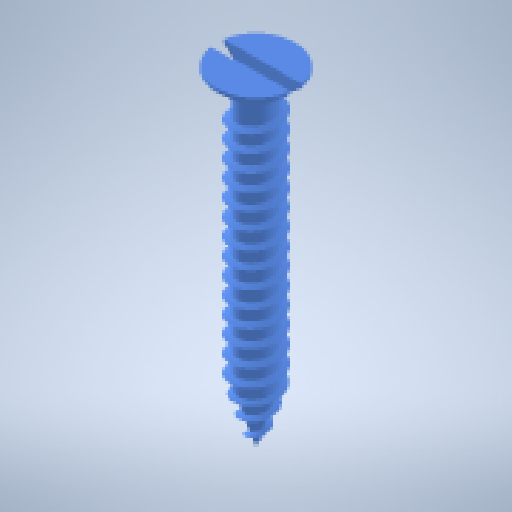
# Autodesk Inventor part: 9 Wood Screw
Saved by Autodesk Inventor 2023 (Build 270158000, 158)
## iProperties
Created: 2023-01-26
Part Number: 9 Wood Screw
Material: Generic
Document SubType Name: Modeling
Designer: 257133
Density: 1 g/cm^3
Appearance: Default
Author: 257133
Autodesk Inventor part; units mm, degrees
ref_plane "XZ Plane" through (0, 0, 0) normal (0, 1, 0) x (-1, 0, 0)
ref_plane "XY Plane" through (0, 0, 0) normal (0, 0, 1) x (1, 0, 0)
sketch "Sketch1" plane through (0, 0, 0) normal (0, 0, 1) x (1, 0, 0)
  line L0 (0, 0) -> (0, 38.1)
  line L1 (0, 38.1) -> (4.572, 38.1)
  line L2 (0, 0) -> (2.0314, 6.35)
  line L3 (0, 0) -> (6.667, 0) construction
  line L4 (2.0314, 6.35) -> (2.0314, 35.5105)
  line L5 (4.572, 38.1) -> (4.572, 37.719)
  line L6 (2.0314, 35.5105) -> (4.572, 37.719)
  line L7 (0, -7.62) -> (0, 45.72) projected
  dimension "d0" = 38.1
  dimension "d1" = 4.572
  dimension "d4" = 0.381
  dimension "d5" = 17.74
  dimension "d6" = 6.35
  dimension "d7" = 41
  dimension "d8" = 2.0314
  constraints: 14 end point, 3 vertical, 2 horizontal, 1 equal length
  measures "d0" distance of L0.start L0.end
  measures "d1" distance of L0.end L1.end
  measures "d4" distance of L1.end L5.end
  measures "d5" angle of L2 L0
  measures "d6" vertical distance of L2.end L0.start
  measures "d7" angle of L6 L1
  measures "d8" distance between parallel lines of L4 L0
revolve "Revolution1" add sketch "Sketch1" angle 360 about axis through (0, -10, 0) along (0, 1, 0)
ref_plane "Work Plane1" through (11.1125, 0, 0) normal (1, 0, 0) x (0, 1, 0)
sketch "Sketch2" plane through (11.1125, 0, 0) normal (1, 0, 0) x (0, 1, 0)
  line L0 (39.4462, 0.762) -> (36.7538, 0.762)
  line L1 (36.7538, 0.762) -> (36.7538, -0.762)
  line L2 (36.7538, -0.762) -> (39.4462, -0.762)
  line L3 (39.4462, -0.762) -> (39.4462, 0.762)
  point P0 (0, 0)
  constraints: 8 end point, 2 parallel, 1 horizontal, 1 perpendicular
extrude "Extrusion1" cut sketch "Sketch2" against normal blind 25.4
sketch "Sketch4" plane through (0, 0, 0) normal (1, 0, 0) x (0, 1, 0)
  line L0 (6.35, -2.0314) -> (6.35, 2.0314) projected
  line L1 (6.35, -2.0314) -> (6.858, -2.0314)
  line L2 (6.858, -2.0314) -> (6.604, -2.7934)
  line L3 (6.604, -2.7934) -> (6.35, -2.0314)
  point P0 (0, 0)
  point P1 (6.604, -2.0314)
  dimension "d19" = 0.508
  dimension "d20" = 0.762
  constraints: 6 end point, 1 equal length, 1 midpoint
  measures "d19" distance of L0.start L1.end
  measures "d20" distance of L2.end point (6.604, -2.031)
coil "Coil1" sketch "Sketch4" operation add axis through (0, -10, 0) along (0, -1, 0) pitch 2.032 turns 3 hand right taper -17.74
coil "Coil2" sketch "Sketch4" operation add axis through (0, -10, 0) along (0, 1, 0) pitch 1.9538 turns 14.3 hand right
body "Solid1"
